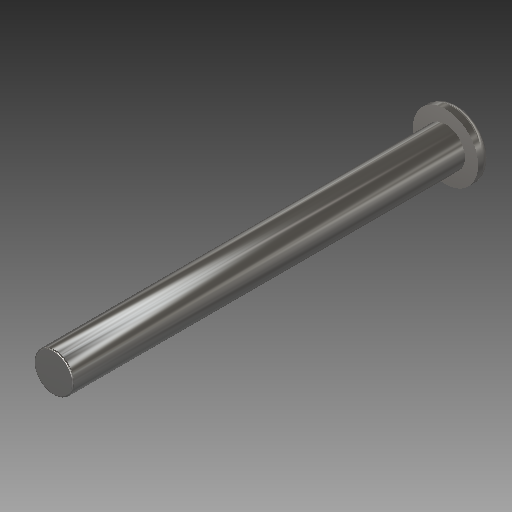
# Autodesk Inventor part: M3-2
Saved by Autodesk Inventor 2017 (Build 210142000, 142)
## iProperties
Created: 2019-12-06
Part Number: M3-2
Material: Generic
Document SubType Name: Modeling
Designer: User
Density: 1 g/cm^3
Appearance: Default
Mass: 0.228196 g
Surface Area: 3.38764 cm^2
Volume: 0.228196 cm^3
Author: User
Autodesk Inventor part; units mm, degrees
ref_plane "YZ Plane" through (0, 0, 0) normal (1, 0, 0) x (0, 1, 0)
ref_plane "XZ Plane" through (0, 0, 0) normal (0, 1, 0) x (-1, 0, 0)
ref_plane "XY Plane" through (0, 0, 0) normal (0, 0, 1) x (1, 0, 0)
sketch "Sketch1" plane through (0, 0, 0) normal (0, 0, 1) x (1, 0, 0)
  circle A0 centre (0, 0) radius 1.5
  dimension "d0" = 3
  constraints: 1 centre point, 1 coincident
  measures "d0" diameter of A0
extrude "Extrusion1" add sketch "Sketch1" along normal blind 30
fillet "Fillet1" radius 0.1 1 edges at (-1.5, 0, 30)
sketch "Sketch2" plane through (0, 0, 0) normal (0, 0, -1) x (-1, 0, 0)
  circle A0 centre (0, 0) radius 2.5
  dimension "d4" = 5
  constraints: 1 centre point, 1 coincident
  measures "d4" diameter of A0
extrude "Extrusion2" add sketch "Sketch2" along normal blind 1
sketch "Sketch3" plane through (0, 0, -1) normal (0, 0, -1) x (-1, 0, 0)
  line L0 (-1.4142, 0.5) -> (1.4142, 0.5)
  line L1 (1.4142, 0.5) -> (1.4142, -0.5)
  line L2 (1.4142, -0.5) -> (-1.4142, -0.5)
  line L3 (-1.4142, -0.5) -> (-1.4142, 0.5)
  line L4 (-1.4142, 0.5) -> (1.4142, -0.5) construction
  line L5 (1.4142, 0.5) -> (-1.4142, -0.5) construction
  line L6 (0.5, 1.4142) -> (-0.5, 1.4142)
  line L7 (-0.5, 1.4142) -> (-0.5, -1.4142)
  line L8 (-0.5, -1.4142) -> (0.5, -1.4142)
  line L9 (0.5, -1.4142) -> (0.5, 1.4142)
  line L10 (0.5, 1.4142) -> (-0.5, -1.4142) construction
  line L11 (-0.5, 1.4142) -> (0.5, -1.4142) construction
  point P0 (0, 0)
  point P1 (0, 0)
  point P2 (0, 0)
  dimension "d8" = 1
  dimension "d9" = 1
  constraints: 24 end point, 4 midpoint, 4 parallel, 2 horizontal, 2 perpendicular
  measures "d8" distance of L0.end L1.end
  measures "d9" distance of L8.end L7.end
extrude "Extrusion3" cut sketch "Sketch3" against normal blind 0.5
fillet "Fillet2" radius 0.6 1 edges at (2.5, 0, -1)
body "Solid1"
